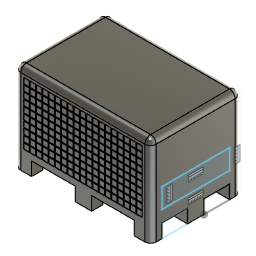
VLOUW Mockup v1 (Autodesk Fusion 360 design; units mm, degrees)
Autodesk Fusion 360 part; units mm, degrees
sketch "Sketch1" plane through (0, 0, 0) normal (0, 0, 1) x (1, 0, 0)
  line L0 (0, 0) -> (1200, 0)
  line L1 (1200, 0) -> (1200, 800)
  line L2 (1200, 800) -> (0, 800)
  line L3 (0, 800) -> (0, 0)
  dimension "d1" = 1200
  dimension "d2" = 800
  constraint horizontal L0
  constraint vertical L1
  constraint horizontal L2
  constraint vertical L3
  constraint coincident L0.start L3.end
  measures "d1" distance of L0.start L0.end
  measures "d2" distance of L0.start L2.end
extrude "Extrude1" add sketch "Sketch1" along normal blind 800
sketch "Sketch2" plane through (1200, 0, 0) normal (1, 0, 0) x (0, 1, 0)
  line L0 (0, 0) -> (800, 0)
  line L1 (800, 0) -> (800, 800)
  line L2 (800, 800) -> (0, 800)
  line L3 (0, 800) -> (0, 0)
  line L4 (100, 0) -> (327.5, 0)
  line L5 (327.5, 0) -> (327.5, 120)
  line L6 (327.5, 120) -> (100, 120)
  line L7 (100, 120) -> (100, 0)
  line L8 (472.4, 0) -> (700, 0)
  line L9 (700, 0) -> (700, 120)
  line L10 (700, 120) -> (472.4, 120)
  line L11 (472.4, 120) -> (472.4, 0)
  dimension "d5" = 100
  dimension "d6" = 227.5
  dimension "d7" = 100
  dimension "d8" = 227.6
  dimension "d9" = 120
  dimension "d10" = 120
  constraint horizontal L4
  constraint vertical L5
  constraint horizontal L6
  constraint vertical L7
  constraint horizontal L8
  constraint vertical L9
  constraint horizontal L10
  constraint vertical L11
  constraint coincident L0 L8.start
  measures "d5" distance of L3 L7
  measures "d6" distance of L5 L7
  measures "d7" distance of L1 L9
  measures "d8" distance of L9 L11
  measures "d9" distance of L4 L6
  measures "d10" distance of L8 L10
extrude "Extrude2" cut sketch "Sketch2" against normal through all contours L0 L4 L5 L6 L7 | L0 L8 L9 L10 L11
fillet "Fillet1" radius 50 7 edges at (600, 0, 800) (0, 400, 800) (600, 800, 800) (1200, 400, 800) (1200, 0, 400) (1200, 800, 400) (0, 0, 400)
fillet "Fillet2" radius 50 2 edges at (0, 800, 375) (14.6447, 785.3553, 785.3553)
sketch "Sketch3" plane through (0, 800, 0) normal (0, 1, 0) x (-1, 0, 0)
  line L0 (-50, 0) -> (-50, 750)
  line L1 (-50, 750) -> (-1150, 750)
  line L2 (-1150, 750) -> (-1150, 0)
  line L3 (-1150, 0) -> (-50, 0)
  line L4 (-1055, 0) -> (-677.7223, 0)
  line L5 (-677.7223, 0) -> (-677.7223, 120)
  line L6 (-677.7223, 120) -> (-1055, 120)
  line L7 (-1055, 120) -> (-1055, 0)
  line L8 (-532.7223, 120) -> (-145, 120)
  line L9 (-145, 120) -> (-145, 0)
  line L10 (-145, 0) -> (-532.7223, 0)
  line L11 (-532.7223, 0) -> (-532.7223, 120)
  dimension "d16" = 120
  dimension "d17" = 120
  dimension "d18" = 145
  dimension "d19" = 95
  dimension "d20" = 95
  constraint horizontal L4
  constraint vertical L5
  constraint horizontal L6
  constraint vertical L7
  constraint coincident L3 L4.start
  constraint horizontal L8
  constraint vertical L9
  constraint horizontal L10
  constraint vertical L11
  constraint coincident L3 L9.end
  measures "d16" distance of L4 L6
  measures "d17" distance of L8 L10
  measures "d18" distance of L5 L11
  measures "d19" distance of L2 L7
  measures "d20" distance of L0 L9
extrude "Extrude3" cut sketch "Sketch3" against normal through all contours L3 L8 L9 L10 L11 | L3 L4 L5 L6 L7
sketch "Sketch4" plane through (0, 800, 0) normal (0, 1, 0) x (-1, 0, 0)
  line L0 (-677.7223, 120) -> (-677.7223, 0)
  line L1 (-677.7223, 0) -> (-532.7223, 0)
  line L2 (-532.7223, 0) -> (-532.7223, 120)
  line L3 (-532.7223, 120) -> (-145, 120)
  line L4 (-145, 120) -> (-145, 0)
  line L5 (-145, 0) -> (-50, 0)
  line L6 (-50, 0) -> (-50, 750)
  line L7 (-50, 750) -> (-1150, 750)
  line L8 (-1150, 750) -> (-1150, 0)
  line L9 (-1150, 0) -> (-1055, 0)
  line L10 (-1055, 0) -> (-1055, 120)
  line L11 (-1055, 120) -> (-677.7223, 120)
  line L12 (-1125, 725) -> (-1075, 725)
  line L13 (-1075, 725) -> (-1075, 675)
  line L14 (-1075, 675) -> (-1125, 675)
  line L15 (-1125, 675) -> (-1125, 725)
  constraint horizontal L12
  constraint vertical L13
  constraint horizontal L14
  constraint vertical L15
extrude "Extrude4" cut sketch "Sketch4" against normal blind 5 contours L12 L13 L14 L15
pattern_linear "R-Pattern1" count 10 spacing 58.3333 along (0, 0, -1) count 19 spacing 55.5556 along (-1, 0, 0) of "Extrude4"
sketch "Sketch5" plane through (0, 0, 0) normal (0, -1, 0) x (1, 0, 0)
  line L0 (677.7223, 0) -> (677.7223, 120)
  line L1 (677.7223, 120) -> (1055, 120)
  line L2 (1055, 120) -> (1055, 0)
  line L3 (1055, 0) -> (1150, 0)
  line L4 (1150, 0) -> (1150, 750)
  line L5 (1150, 750) -> (50, 750)
  line L6 (50, 750) -> (50, 0)
  line L7 (50, 0) -> (145, 0)
  line L8 (145, 0) -> (145, 120)
  line L9 (145, 120) -> (532.7223, 120)
  line L10 (532.7223, 120) -> (532.7223, 0)
  line L11 (532.7223, 0) -> (677.7223, 0)
  line L12 (75, 725) -> (125, 725)
  line L13 (125, 725) -> (125, 675)
  line L14 (125, 675) -> (75, 675)
  line L15 (75, 675) -> (75, 725)
  constraint horizontal L12
  constraint vertical L13
  constraint horizontal L14
  constraint vertical L15
extrude "Extrude5" cut sketch "Sketch5" against normal blind 3 contours L12 L13 L14 L15
pattern_linear "R-Pattern2" count 10 spacing 55.5556 along (0, 0, -1) count 19 spacing 55.5556 along (1, 0, 0) of "Extrude5"
sketch "Sketch7" plane through (1200, 0, 0) normal (1, 0, 0) x (0, 1, 0)
  line L0 (100, 400) -> (700, 400)
  line L1 (700, 400) -> (700, 225)
  line L2 (700, 225) -> (100, 225)
  line L3 (100, 225) -> (100, 400)
  constraint horizontal L0
  constraint vertical L1
  constraint horizontal L2
  constraint vertical L3
